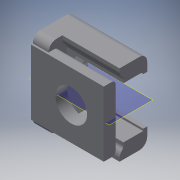
# Autodesk Inventor part: nut holder
Saved by Autodesk Inventor 2016 (Build 200138000, 138)
## iProperties
Created: 2016-02-14
Part Number: nut holder
Material: Generic
Document SubType Name: Modeling
Designer: Erwin
Density: 1 g/cm^3
Appearance: Default
Author: Erwin
Autodesk Inventor part; units mm, degrees
ref_plane "YZ Plane" through (0, 0, 0) normal (1, 0, 0) x (0, 1, 0)
ref_plane "XZ Plane" through (0, 0, 0) normal (0, 1, 0) x (-1, 0, 0)
ref_plane "XY Plane" through (0, 0, 0) normal (0, 0, 1) x (1, 0, 0)
sketch "Sketch1" plane through (0, 0, 0) normal (0, 1, 0) x (-1, 0, 0)
  line L0 (0, 0) -> (16.5, 0)
  line L1 (16.5, 0) -> (16.5, -16.5)
  line L2 (16.5, -16.5) -> (0, -16.5)
  line L3 (0, -16.5) -> (0, 0)
  dimension "d0" = 16.5
  dimension "d1" = 16.5
  constraints: 8 end point, 2 parallel, 1 horizontal, 1 perpendicular
  measures "d0" distance of L1.end L2.end
  measures "d1" distance of L0.end L1.end
extrude "Extrusion1" add sketch "Sketch1" along normal blind 11
sketch "Sketch2" plane through (0, 0, 0) normal (1, 0, 0) x (0, 0, -1)
  line L0 (0, 0) -> (0, 5)
  line L1 (1, 6) -> (15.5, 6)
  line L2 (16.5, 0) -> (16.5, 11) projected
  line L3 (16.5, 0) -> (16.5, 5)
  arc A0 (1, 6) -> (0, 5) centre (1, 5) ccw
  arc A1 (16.5, 5) -> (15.5, 6) centre (15.5, 5) ccw
  line L4 (0, 5) -> (0, 6)
  line L5 (1, 7) -> (15.5, 7)
  line L6 (16.5, 5) -> (16.5, 6)
  arc A2 (1, 7) -> (0, 6) centre (1, 6) ccw
  arc A3 (16.5, 6) -> (15.5, 7) centre (15.5, 6) ccw
  line L7 (0, 11) -> (16.5, 11) projected
  line L8 (16.5, 11) -> (0, 11) projected
  point P0 (0, 6)
  point P1 (16.5, 6)
  point P2 (0, 7)
  point P3 (16.5, 7)
  dimension "d4" = 6
  dimension "d5" = 1
  dimension "d6" = 2
  dimension "d7" = 1
  constraints: 12 end point, 10 point on line, 8 point on circle, 8 tangent, 4 centre point, 2 collinear, 2 equal radius, 2 perpendicular, 2 vertical
  measures "d4" distance of L0.start point (0, 6)
  measures "d5" radius of A0
  measures "d6" distance of L0.end point (0, 7)
  measures "d7" radius of A2
sketch "Sketch3" plane through (0, 11, 0) normal (0, 1, 0) x (1, 0, 0)
  line L0 (-15.7556, 8.25) -> (-12.0028, 14.75)
  line L1 (-12.0028, 14.75) -> (-4.4972, 14.75)
  line L2 (-4.4972, 14.75) -> (-0.7444, 8.25)
  line L3 (-0.7444, 8.25) -> (-4.4972, 1.75)
  line L4 (-4.4972, 1.75) -> (-12.0028, 1.75)
  line L5 (-12.0028, 1.75) -> (-15.7556, 8.25)
  point P0 (0, 0)
  point P1 (-8.25, 8.25)
  dimension "d8" = 13
  constraints: 12 end point, 13 other
  measures "d8" distance between parallel lines of L1 L4
extrude "Extrusion2" cut sketch "Sketch3" against normal blind 5
sketch "Sketch4" plane through (0, 6, 0) normal (0, 1, 0) x (1, 0, 0)
  line L0 (-4.4972, 1.75) -> (-12.0028, 1.75) projected
  line L1 (-12.0028, 14.75) -> (-4.4972, 14.75) projected
  circle A0 centre (-8.25, 8.25) radius 4
  point P0 (0, 0)
  dimension "d11" = 8
  constraints: 1 centre point
  measures "d11" diameter of A0
extrude "Extrusion3" cut sketch "Sketch4" against normal blind 20
extrude "Extrusion4" cut sketch "Sketch2" against normal blind 12.5
sketch "Sketch5" plane through (0, 11, 0) normal (0, 1, 0) x (1, 0, 0)
  line L0 (-4.4972, 1.75) -> (-12.0028, 1.75) projected
  line L1 (-12.0028, 1.75) -> (3.1486, 1.75)
  line L2 (3.1486, 1.75) -> (3.1486, 14.75)
  line L3 (3.1486, 14.75) -> (-12.0028, 14.75)
  line L4 (-12.0028, 14.75) -> (-12.0028, 1.75)
  point P0 (0, 0)
  dimension "d16" = 13
  constraints: 8 end point, 2 parallel, 1 horizontal, 1 perpendicular
  measures "d16" distance of L2.end L1.end
extrude "Extrusion5" cut sketch "Sketch5" against normal up to surface (4 mm away)
sketch "Sketch6" plane through (-16.5, 0, -16.5) normal (-1, 0, 0) x (0, 0, 1)
  line L0 (16.5, 0) -> (0, 0) projected
  line L1 (16.5, 0) -> (16.5, 11) projected
  line L2 (0, 11) -> (16.5, 11) projected
  line L3 (0, 0) -> (0, 11) projected
extrude "Extrusion6" add sketch "Sketch6" along normal blind 2
sketch "Sketch7" plane through (0, 0, 0) normal (0, -1, 0) x (1, 0, 0)
  circle A0 centre (-8.25, -8.25) radius 4 projected
  line L0 (0, 0) -> (-18.5, 0) projected
  line L1 (-18.5, -16.5) -> (-18.5, 0) projected
  line L2 (-18.5, -16.5) -> (0, -16.5) projected
  line L3 (0, -16.5) -> (0, 0) projected
extrude "Extrusion7" cut sketch "Sketch7" against normal blind 1
sketch "Sketch8" plane through (0, 11, 0) normal (0, 1, 0) x (1, 0, 0)
  line L0 (0, 1.75) -> (-12.0028, 1.75) projected
  line L1 (-12.0028, 1.75) -> (-15.7556, 8.25) projected
  line L2 (-15.7556, 8.25) -> (-12.0028, 14.75) projected
  line L3 (-12.0028, 14.75) -> (0, 14.75) projected
  line L4 (0, 14.75) -> (0, 16.5) projected
  line L5 (0, 16.5) -> (-18.5, 16.5) projected
  line L6 (-18.5, 0) -> (-18.5, 16.5) projected
  line L7 (0, 0) -> (-18.5, 0) projected
  line L8 (0, 0) -> (0, 1.75) projected
extrude "Extrusion8" add sketch "Sketch8" along normal blind 3
sketch "Sketch10" plane through (0, 7, -1) normal (1, 0, 0) x (0, 0, -1)
  line L0 (15.5, -1) -> (15.5, -2) projected
  line L1 (15.5, -1) -> (-1, -1)
  line L2 (-1, -1) -> (-1, 0)
  line L3 (0, 1) -> (14.5, 1)
  line L4 (15.5, 0) -> (15.5, -1)
  arc A0 (0, 1) -> (-1, 0) centre (0, 0) ccw
  arc A1 (15.5, 0) -> (14.5, 1) centre (14.5, 0) ccw
  point P0 (-1, -7)
  point P1 (-1, 1)
  point P2 (15.5, 1)
  dimension "d28" = 16.5
  dimension "d29" = 2
  dimension "d30" = 1
  constraints: 8 end point, 4 point on circle, 4 point on line, 4 tangent, 2 centre point, 2 parallel, 1 equal radius, 1 horizontal, 1 perpendicular
  measures "d28" distance of point (-1, 1) point (15.5, 1)
  measures "d29" distance of L1.end point (-1, 1)
  measures "d30" radius of A0
extrude "Extrusion9" cut sketch "Sketch10" against normal up to surface (12.5 mm away)
sketch "Sketch11" plane through (0, 5, -16.5) normal (0, 0, -1) x (-1, 0, 0)
  line L0 (18.5, 9) -> (0, 9) projected
  line L1 (0, 2) -> (0, 9) projected
  line L2 (18.5, 9) -> (0, 9)
  line L3 (0, 9) -> (0, 2)
  line L4 (0, 2) -> (18.5, 2)
  line L5 (18.5, 2) -> (18.5, 9)
  point P0 (0, -5)
  constraints: 8 end point, 2 parallel, 1 horizontal, 1 perpendicular
extrude "Extrusion10" add sketch "Sketch11" along normal blind 2
ref_plane "Work Plane1" through (-15.7556, 14, -8.25) normal (0, 0, -1) x (-1, 0, 0)
mirror "Mirror1" about plane through (-15.7556, 14, -8.25) normal (0, 0, -1) of "Extrusion8", "Extrusion10", "Extrusion9", "Extrusion2"
sketch "Sketch12" plane through (-18.5, 0, -16.5) normal (-1, 0, 0) x (0, 0, 1)
  line L0 (18.5, 14) -> (18.5, 7) projected
  line L1 (18.5, 10.5) -> (-2, 10.5)
  line L2 (-2, 10.5) -> (-2, 3.5)
  line L3 (-2, 3.5) -> (18.5, 3.5)
  line L4 (18.5, 3.5) -> (18.5, 10.5)
  point P0 (16.5, 0)
  point P1 (18.5, 11)
  point P2 (18.5, 9)
  constraints: 8 end point, 2 parallel, 1 horizontal, 1 midpoint, 1 perpendicular
extrude "Extrusion11" add sketch "Sketch12" against normal up to surface (6 mm away)
fillet "Fillet3" radius 2 2 edges at (-15.5, 3.5, -18.5) (-15.5, 3.5, 2)
fillet "Fillet4" radius 2 2 edges at (-9.25, 14, -18.5) (-9.25, 14, 2)
fillet "Fillet5" radius 2 2 edges at (-6.25, 7, -16.5) (-6.25, 7, 0)
sketch "Sketch13" plane through (-12.5, 10.5, -2.6112) normal (0, 1, 0) x (1, 0, 0)
  line L0 (-3.2556, 5.6388) -> (0, 11.2776) projected
  line L1 (0, 0) -> (-3.2556, 5.6388) projected
  line L2 (0, 0) -> (0, 11.2776) projected
  point P0 (12.5, -2.6112)
extrude "Extrusion12" cut sketch "Sketch13" against normal blind 3
sketch "Sketch14" plane through (-12.5, 0, 0) normal (1, 0, 0) x (0, 0, -1)
  line L0 (13.8888, 8) -> (13.8888, 7.5) projected
  line L1 (13.8888, 7.5) -> (2.6112, 7.5) projected
  line L2 (2.6112, 7.5) -> (2.6112, 8) projected
  line L3 (1, 8) -> (2.6112, 8) projected
  arc A0 (1, 8) -> (0.2546, 7.6667) centre (1, 7) ccw projected
  arc A1 (-1.2361, 7) -> (0.2546, 7.6667) centre (-1.2361, 9) ccw projected
  line L4 (-2, 7) -> (-1.2361, 7) projected
  line L5 (-2, 5.5) -> (-2, 7) projected
  arc A2 (-2, 5.5) -> (0, 3.5) centre (0, 5.5) ccw projected
  line L6 (0, 5) -> (0, 3.5) projected
  arc A3 (1, 6) -> (0, 5) centre (1, 5) ccw projected
  line L7 (15.5, 6) -> (1, 6) projected
  arc A4 (16.5, 5) -> (15.5, 6) centre (15.5, 5) ccw projected
  line L8 (16.5, 3.5) -> (16.5, 5) projected
  arc A5 (16.5, 3.5) -> (18.5, 5.5) centre (16.5, 5.5) ccw projected
  line L9 (18.5, 7) -> (18.5, 5.5) projected
  line L10 (17.7361, 7) -> (18.5, 7) projected
  arc A6 (16.2454, 7.6667) -> (17.7361, 7) centre (17.7361, 9) ccw projected
  arc A7 (16.2454, 7.6667) -> (15.5, 8) centre (15.5, 7) ccw projected
  line L11 (13.8888, 8) -> (15.5, 8) projected
  line L12 (13.8888, 8) -> (2.6112, 8)
  line L13 (2.6112, 8) -> (2.6112, 7.5)
  line L14 (2.6112, 7.5) -> (13.8888, 7.5)
  line L15 (13.8888, 7.5) -> (13.8888, 8)
  point P0 (0, 0)
  constraints: 8 end point, 2 parallel, 1 horizontal, 1 perpendicular
extrude "Extrusion13" cut sketch "Sketch14" against normal blind 2
sketch "Sketch15" plane through (0, 14, 0) normal (0, 1, 0) x (1, 0, 0)
  line L0 (0, 0) -> (-18.5, 0) projected
  line L1 (0, 1.75) -> (0, 0) projected
  line L2 (0, 1.75) -> (-12.0028, 1.75) projected
  line L3 (-12.0028, 1.75) -> (-15.7556, 8.25) projected
  line L4 (-15.7556, 8.25) -> (-12.0028, 14.75) projected
  line L5 (-12.0028, 14.75) -> (0, 14.75) projected
  line L6 (0, 14.75) -> (0, 16.5) projected
  line L7 (-18.5, 16.5) -> (0, 16.5) projected
  line L8 (-18.5, 0) -> (-18.5, 16.5) projected
  line L9 (-11.7141, 14.25) -> (-15.1782, 8.25)
  line L10 (-15.1782, 8.25) -> (-11.7141, 2.25)
  line L11 (-11.7141, 2.25) -> (0, 2.25)
  line L12 (0, -0.5) -> (-19, -0.5)
  line L13 (-19, -0.5) -> (-19, 17)
  line L14 (-19, 17) -> (0, 17)
  line L15 (0, 14.25) -> (-11.7141, 14.25)
  line L16 (0, 14.75) -> (0, 14.25)
  line L17 (0, 2.25) -> (0, 1.75)
  line L18 (0.5, 2.25) -> (0.5, 1.75)
  line L19 (0.5, 14.75) -> (0.5, 14.25)
  point P0 (0, 0)
  dimension "d45" = 0.5
  constraints: 22 end point, 4 point on line, 2 vertical, 1 other
  measures "d45" distance between parallel lines of L4 L9
extrude "Extrusion14" add sketch "Sketch15" against normal blind 1 contours L2 L3 L4 L5 L16 L15 L9 L10 L11 L17
move or copy body "Move Body1" bodies to move or copy 1 copy no translate (0, 2, 0)
body "Solid1"
